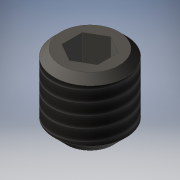
# Autodesk Inventor part: 60199320_4
Saved by Autodesk Inventor 2019 (Build 230136000, 136)
## iProperties
Created: 2024-03-16
Part Number: 60199320_4
Material: Generic
Catalog Web Link: www.cadenas.de
Description: gew-stift_kpl_hzd_rf-Hexagon Socket Set Screws, Torsionally-Stiff Couplings HZD with Through Holes, Stainless, Set-screw style
Vendor: MAEDLER
Document SubType Name: Modeling
Designer: psAdmin
Manufacturer: MAEDLER
Mass: 0.323254 g
Surface Area: 3.10799 cm^2
Volume: 0.323254 cm^3
Density: 1 g/cm^3
Appearance: PSOLRGB-222-219-214
Category: PARTsolutions
Company: MAEDLER
Title: 60199320
Author: Cadenas PARTsolutions
Comments: Hexagon Socket Set Screws, Torsionally-Stiff Couplings HZD with Through Holes, Stainless, Set-screw style
PSOL_IDENT_0: {$CADENAS_DATA/23d-libs/maedler/antriebselemente/kupplungen/drehstarre_kupplungen/dr_k_hzd_m_db_rf/g
PSOL_IDENT_1: ew-stift_kpl_hzd_rf.prj},173 {VTYP=3D},{NB=60199320_4},{LINA=60199320},{NN=gew-stift_kpl_hzd_rf},{DA
PSOL_IDENT_2: TE=09.12.2023 00:25:53},{GEOMDATE=01.12.2023 07:25:45},{VERSION=},{LINEID=320},{WBVAR=},{WBNUMERIC=}
PSOL_IDENT_3: {NB=60199320_4},{LINA=60199320},{KT=DUMMY},{ARTNR=60199320},{WEBSHOP=Produktdetails / Katalogseite
PSOL_IDENT_4: / Montageanleitung},{MATK=Edelstahl},{MAT=Naben aus Edelstahl rostfrei 1.4305 (V2A), Übertragungsel
PSOL_IDENT_5: ement (Kreuzscheibe) aus schwarzem Polyacetal},{D=M8},{L=8},{DZMIN=4.70},{DZMAX=5.0},{S=4.0},{GEW=1.
PSOL_IDENT_6: 880},{DD=8},{T=3.0},{D3=6.77},{G=90},{TN=gew-stift_kpl_hzd_rf_50.0_20},{CTN=84836080}
NB: 60199320_4
NN: gew-stift_kpl_hzd_rf
NT: Hexagon Socket Set Screws, Torsionally-Stiff Couplings HZD with Through Holes, Stainless, Set-screw style
NBSYN: $ARTNR._4
LINA: 60199320
CATALOG: Mädler
ARTNR: 60199320
WEBSHOP: Produktdetails / Katalogseite / Montageanleitung
MATK: Edelstahl
MAT: Naben aus Edelstahl rostfrei 1.4305 (V2A), Übertragungselement (Kreuzscheibe) aus schwarzem Polyacetal
D: M8
L: 8
DZMIN: 4.7
DZMAX: 5
S: 4
GEW: 1.88
DD: 8
T: 3
D3: 6.77
G: 90
TN: gew-stift_kpl_hzd_rf_50.0_20
CTN: 84836080
SUPPLIER: MAEDLER
ARTICLENO: 60199320_4
BOMINFO: 60199320
CREATOR: CADENAS GmbH
Autodesk Inventor part; units mm, degrees
ref_plane "YZ Plane" through (0, 0, 0) normal (1, 0, 0) x (0, 1, 0)
ref_plane "XZ Plane" through (0, 0, 0) normal (0, 1, 0) x (-1, 0, 0)
ref_plane "XY Plane" through (0, 0, 0) normal (0, 0, 1) x (1, 0, 0)
sketch "Sketch_1" plane through (0, 0, 0) normal (0, 0, 1) x (1, 0, 0)
  line L0 (0, -6.5999) -> (0, 0)
  line L1 (0, 0) -> (3.233, 0)
  line L2 (3.233, 0) -> (4, -0.767)
  line L3 (4, -0.767) -> (4, -8)
  line L4 (4, -8) -> (2.425, -8)
  line L5 (2.425, -8) -> (0, -6.5999)
  line L6 (0, -6.5999) -> (0, 0)
  constraints: 14 end point
revolve "Revolution1" add sketch "Sketch_1" angle 360 about axis through (0, -6.5999, 0) along (0, -1, 0)
thread "Thread1" size "M8x1.25" class "6g" standard "ISO Metric profile" full length
sketch "Sketch_7" plane through (0, 0, 0) normal (0, 0, 1) x (1, 0, 0)
  line L0 (0, -50) -> (0, 50)
  line L1 (2.5999, -8) -> (8, -8)
  line L2 (8, -8) -> (8, -6.5999)
  line L3 (8, -6.5999) -> (4, -6.5999)
  line L4 (4, -6.5999) -> (2.5999, -8)
  constraints: 10 end point
revolve "Revolution2" cut sketch "Sketch_7" angle 360 about axis through (0, -50, 0) along (0, -1, 0)
sketch "Sketch_2" plane through (0, 0, 0) normal (0, 1, 0) x (-1, 0, 0)
  line L0 (2, 1.1547) -> (0, 2.3094)
  line L1 (0, 2.3094) -> (-2, 1.1547)
  line L2 (-2, 1.1547) -> (-2, -1.1547)
  line L3 (-2, -1.1547) -> (0, -2.3094)
  line L4 (0, -2.3094) -> (2, -1.1547)
  line L5 (2, -1.1547) -> (2, 1.1547)
  constraints: 12 end point
extrude "Extrusion1" cut sketch "Sketch_2" against normal blind 3
ref_plane "gew_stift_XY" through (0, 0, 0) normal (0, 1, 0) x (1, 0, 0)
ref_plane "gew_stift_YZ" through (0, 0, 0) normal (1, 0, 0) x (0, 0, -1)
ref_plane "gew_stift_ZX" through (0, 0, 0) normal (0, 0, -1) x (0, 1, 0)
body "Solid1"
